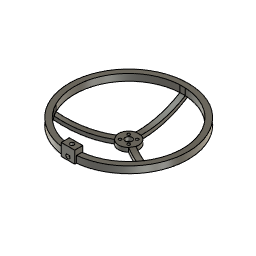
Frame_Prop_4 v5 (Autodesk Fusion 360 design; units mm, degrees)
Autodesk Fusion 360 part; units mm, degrees
note: some values were not read from the file. Set by a fixed rule: which face or edge a step refers to.
sketch "スケッチ1" plane through (0, 0, 0) normal (0, 0, 1) x (1, 0, 0)
  circle A0 centre (0, 0) radius 44
  circle A1 centre (0, 0) radius 40
  dimension "d1" = 88
  dimension "d2" = 80
  constraint coincident A0.centre A1.centre
  constraint concentric A0 A1
  measures "d1" diameter of A0
  measures "d2" diameter of A1
extrude "押し出し1" add sketch "スケッチ1" along normal blind 5 makes body 1
sketch "スケッチ2" plane through (0, 0, 5) normal (0, 0, 1) x (-1, 0, 0)
  circle A0 centre (0, 0) radius 40
  circle A1 centre (0, 0) radius 44
  line L0 (0, 44) -> (0, 40)
  line L1 (-5, 45) -> (5, 45)
  line L2 (5, 45) -> (5, 39)
  line L3 (5, 39) -> (-5, 39)
  line L4 (-5, 39) -> (-5, 45)
  line L5 (-5, 45) -> (5, 39) construction
  line L6 (5, 45) -> (-5, 39) construction
  point P0 (0, 42)
  dimension "d5" = 10
  dimension "d6" = 6
  constraint coincident A1 L0.start
  constraint coincident A0 L0.end
  constraint horizontal L1
  constraint perpendicular L1 L2
  constraint parallel L1 L3
  constraint parallel L2 L4
  constraint coincident L5 P0
  constraint coincident L6 P0
  constraint midpoint L0 P0
  measures "d5" distance of L2.end L3.end
  measures "d6" distance of L1.end L2.end
extrude "押し出し2" add sketch "スケッチ2" along normal blind 4 and the other way blind 5 contours A0 L2 L3 L4 | A0 A1 L0 L2 | A0 A1 L0 L4 | A1 L1 L2 L4 picked at (0, 39.3333) bodies 1
sketch "スケッチ3" plane through (0, -45, 0) normal (0, -1, 0) x (1, 0, 0)
  line L0 (5, 0) -> (5, 9)
  line L1 (5, 9) -> (-5, 9)
  line L2 (-5, 9) -> (-5, 0)
  line L3 (-5, 0) -> (5, 0)
  line L4 (0, 0) -> (0, 2.5)
  circle A0 centre (0, 2.5) radius 1.55
  dimension "d11" = 2.5
  dimension "d12" = 3.1
  constraint coincident L4.start origin
  constraint perpendicular L3 L4
  constraint coincident L4.end A0.centre
  measures "d11" distance of L4.start L4.end
  measures "d12" diameter of A0
extrude "押し出し3" cut sketch "スケッチ3" against normal blind 10 contours A0 bodies 1
sketch "スケッチ4" plane through (0, -45, 0) normal (0, -1, 0) x (1, 0, 0)
  circle A0 centre (0, 2.5) radius 1.55
  line L0 (5, 0) -> (5, 9)
  line L1 (5, 9) -> (-5, 9)
  line L2 (-5, 9) -> (-5, 0)
  line L3 (-5, 0) -> (5, 0)
  circle A1 centre (0, 2.5) radius 1.55
  line L4 (0, 4.05) -> (0, 3.55)
  line L5 (-1.1402, 3.55) -> (1.1402, 3.55)
  dimension "d15" = 0.5
  constraint concentric A0 A1
  constraint coincident A0 L4.start
  constraint vertical L4
  constraint coincident A1 L5.start
  constraint coincident A1 L5.end
  constraint perpendicular L4 L5
  measures "d15" distance of L4.start L4.end
extrude "押し出し4" add sketch "スケッチ4" against normal blind 6 contours A0 A1 L4 L5 | A0 A1 L4 L5 bodies 1
sketch "スケッチ5" plane through (0, 0, 9) normal (0, 0, 1) x (-1, 0, 0)
  line L0 (-5, 39) -> (5, 39)
  line L1 (5, 39) -> (5, 45)
  line L2 (5, 45) -> (-5, 45)
  line L3 (-5, 45) -> (-5, 39)
  line L4 (0, 39) -> (0, 42)
  circle A0 centre (0, 42) radius 1.45
  dimension "d18" = 3
  dimension "d19" = 2.9
  constraint midpoint L0 L4.start
  constraint perpendicular L2 L4
  constraint coincident L4.end A0.centre
  measures "d18" distance of L4.start L4.end
  measures "d19" diameter of A0
extrude "押し出し5" cut sketch "スケッチ5" against normal blind 9 contours A0 bodies 1
sketch "スケッチ6" plane through (0, 0, 5) normal (0, 0, 1) x (-1, 0, 0)
  line L0 (-5, 39.6863) -> (-5, 43.715)
  arc A0 (-5, 43.715) -> (5, 43.715) centre (0, 0) ccw
  line L1 (5, 43.715) -> (5, 39.6863)
  arc A1 (-5, 39.6863) -> (5, 39.6863) centre (0, 0) ccw
  circle A2 centre (0, 0) radius 7.5
  dimension "d22" = 15
  constraint concentric A0 A2
  measures "d22" diameter of A2
extrude "押し出し6" add sketch "スケッチ6" against normal blind 17 separate body contours A2 makes body 2
extrude "押し出し7" cut 1 faces at (-1.9158, -2.8099, 5) along direction (0, 0, -1) blind 14 on bodies 2 bodies 2
sketch "スケッチ7" plane through (0, 0, -9) normal (0, 0, 1) x (-1, 0, 0)
  circle A0 centre (0, 0) radius 7.5
  circle A1 centre (0, 0) radius 2.5
  line L0 (0, 0) -> (3.182, 3.182)
  line L1 (0, 0) -> (4.5, 0) construction
  circle A2 centre (3.182, 3.182) radius 1
  circle A3 centre (-3.182, 3.182) radius 1
  circle A4 centre (-3.182, -3.182) radius 1
  circle A5 centre (3.182, -3.182) radius 1
  dimension "d27" = 5
  dimension "d28" = 4.5
  dimension "d29" = 45
  dimension "d30" = 2
  dimension "d32" = 360
  constraint concentric A0 A1
  constraint horizontal L1
  constraint coincident A0.centre A1.centre
  constraint coincident L0.end A2.centre
  measures "d27" diameter of A1
  measures "d28" distance of A0.centre L0.end
  measures "d29" angle of L0 L1
  measures "d30" diameter of A2
extrude "押し出し8" cut sketch "スケッチ7" against normal blind 3 contours A1 | A2 | A3 | A4 | A5 bodies 2
sketch "スケッチ8" plane through (0, 0, 5) normal (0, 0, 1) x (-1, 0, 0)
  line L0 (-5, 39.6863) -> (-5, 43.715)
  arc A0 (-5, 43.715) -> (5, 43.715) centre (0, 0) ccw
  line L1 (5, 43.715) -> (5, 39.6863)
  arc A1 (-5, 39.6863) -> (5, 39.6863) centre (0, 0) ccw
  circle A2 centre (0, 0) radius 2.5
  circle A3 centre (-3.182, -3.182) radius 1
  circle A4 centre (-3.182, 3.182) radius 1
  circle A5 centre (3.182, -3.182) radius 1
  circle A6 centre (3.182, 3.182) radius 1
  circle A7 centre (0, 0) radius 7.5
  line L2 (0, 0) -> (-2, 0)
  line L3 (-2, 0) -> (2, 0)
  line L4 (2, 0) -> (2, -43.9545)
  line L5 (2, -43.9545) -> (-2, -43.9545)
  line L6 (-2, -43.9545) -> (-2, 0)
  line L7 (39.0657, 20.2452) -> (1, -1.7321)
  line L8 (-1, 1.7321) -> (37.0657, 23.7093)
  line L9 (1, -1.7321) -> (-1, 1.7321)
  line L10 (37.0657, 23.7093) -> (39.0657, 20.2452)
  line L11 (-37.0657, 23.7093) -> (1, 1.7321)
  line L12 (-1, -1.7321) -> (-39.0657, 20.2452)
  line L13 (1, 1.7321) -> (-1, -1.7321)
  line L14 (-39.0657, 20.2452) -> (-37.0657, 23.7093)
  dimension "d35" = 2
  dimension "d36" = 4
  dimension "d38" = 360
  constraint coincident A0.centre A1.centre
  constraint horizontal L2
  constraint horizontal L3
  constraint vertical L4
  constraint horizontal L5
  constraint vertical L6
  constraint coincident A0 L4.end
  measures "d35" distance of A0.centre L2.end
  measures "d36" distance of L2.end L3.end
extrude "押し出し9" add sketch "スケッチ8" against normal blind 17 contours A1 A7 L11 L12 | A1 L11 L12 L14 | A0 L14 | A1 A7 L4 L6 | A1 L4 L5 L6 | A1 A7 L7 L8 | A0 L5 | A1 L7 L8 L10 | A0 L10 bodies 1 2
sketch "スケッチ9" plane through (1, -1.7321, 0) normal (0.5, -0.866025, 0) x (0.866025, 0.5, 0)
  line L0 (-39.95, 5) -> (-39.95, 0)
  line L1 (-39.95, 0) -> (-43.9545, 0)
  line L2 (-43.9545, 0) -> (-43.9545, -12)
  line L3 (-43.9545, -12) -> (-7.2284, -12)
  line L4 (-7.2284, -12) -> (-7.2284, -9)
  line L5 (-7.2284, -9) -> (-7.2284, 5)
  line L6 (-7.2284, 5) -> (-39.95, 5)
  arc A0 (-43.9545, 0) -> (-7.2284, -12) centre (-7.2284, 50.2003) ccw
  arc A1 (-39.95, 0) -> (-7.2284, -9) centre (-8.1735, 51.5474) ccw
  constraint tangent L3 A0
  constraint coincident L1.end L2.start
  constraint coincident L3.end L4.start
  constraint tangent A0 A1
  constraint coincident L0.end L1.start
  constraint coincident L4.end L5.start
extrude "押し出し10" cut sketch "スケッチ9" against normal blind 4 contours L0 L5 L6 A1 | L2 L3 A0 bodies 1
pattern_circular "C パターン1" count 3 over 360 about axis through (0, 0, 1.75) along (0, 0, 1) of "押し出し10"
extrude "押し出し11" cut 3 faces at (-38.1885, -21.7915, -12) (37.9663, -22.1765, -12) (0.2223, 43.968, -12) along direction (0, 0, 1) blind 12 on bodies 1 bodies 1
